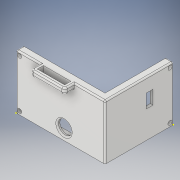
# Autodesk Inventor part: Part1
Saved by Autodesk Inventor 2019 (Build 230136000, 136)
## iProperties
Created: 2019-02-07
Part Number: Part1
Material: ABS Plastic
Document SubType Name: Modeling
Designer: darky
Density: 1.06 g/cm^3
Appearance: Smooth - White
Author: darky
Autodesk Inventor part; units mm, degrees
ref_plane "YZ Plane" through (0, 0, 0) normal (1, 0, 0) x (0, 1, 0)
ref_plane "XZ Plane" through (0, 0, 0) normal (0, 1, 0) x (-1, 0, 0)
ref_plane "XY Plane" through (0, 0, 0) normal (0, 0, 1) x (1, 0, 0)
sketch "Sketch1" plane through (0, 0, 0) normal (0, 0, 1) x (1, 0, 0)
  line L0 (0, 0) -> (65, 0)
  line L1 (65, 0) -> (65, 40)
  line L2 (65, 40) -> (0, 40)
  line L3 (0, 40) -> (0, 0)
  dimension "d0" = 65
  dimension "d1" = 40
  constraints: 8 end point, 2 parallel, 1 horizontal, 1 perpendicular
  measures "d0" distance of L2.end L1.end
  measures "d1" distance of L1.end L0.end
extrude "Extrusion1" add sketch "Sketch1" along normal blind 50
shell "Shell1" thickness 5 removed faces 4 at (43.3333, 40, 16.6667) at (21.6667, 13.3333, 0) at (0, 26.6667, 16.6667) at (21.6667, 0, 16.6667)
sketch "Sketch4" plane through (0, 0, 50) normal (0, 0, 1) x (1, 0, 0)
  line L0 (65, 0) -> (65, 40) projected
  line L1 (65, 0) -> (35, 0)
  line L2 (0, 0) -> (65, 0) projected
  line L3 (35, 0) -> (35, 8)
  circle A0 centre (35, 8) radius 5
  dimension "d17" = 30
  dimension "d18" = 8
  dimension "d19" = 10
  constraints: 4 end point, 1 centre point, 1 coincident, 1 perpendicular, 1 point on line
  measures "d17" distance of L0.start L1.end
  measures "d18" distance of L1.end L3.end
  measures "d19" diameter of A0
extrude "Extrusion4" cut sketch "Sketch4" against normal blind 3
sketch "Sketch5" plane through (0, 0, 50) normal (0, 0, 1) x (1, 0, 0)
  point P0 (0, 0)
sketch "Sketch6" plane through (35, 8, 47) normal (0, 0, 1) x (1, 0, 0)
  circle A0 centre (0, 0) radius 3
  point P0 (-35, -8)
  dimension "d22" = 6
  constraints: 1 centre point
  measures "d22" diameter of A0
extrude "Extrusion5" cut sketch "Sketch6" against normal blind 2
sketch "Sketch7" plane through (0, 0, 50) normal (0, 0, 1) x (1, 0, 0)
  line L0 (0, 0) -> (65, 0) projected
  line L1 (0, 0) -> (5, 0)
  line L2 (5, 0) -> (5, 5)
  line L3 (65, 40) -> (0, 40) projected
  line L4 (5, 5) -> (5, 35)
  line L5 (5, 35) -> (2.5, 37.4495)
  circle A0 centre (2.5, 37.4495) radius 1.9
  dimension "d25" = 5
  dimension "d26" = 5
  dimension "d27" = 30
  dimension "d28" = 3.5
  dimension "d29" = 3.8
  constraints: 8 end point, 2 point on line, 1 centre point, 1 coincident, 1 perpendicular
  measures "d25" distance of L0.start L1.end
  measures "d26" distance of L1.end L2.end
  measures "d27" distance of L2.end L4.end
  measures "d28" distance of L4.end L5.end
  measures "d29" diameter of A0
hole "Hole1" at (2.5, 37.4495, 50) direction (0, 0, -1) diameter 3 depth 9 tip angle 118
sketch "Sketch8" plane through (0, 0, 50) normal (0, 0, 1) x (1, 0, 0)
  line L0 (0, 0) -> (5, 0)
  line L1 (0, 0) -> (65, 0) projected
  line L2 (5, 0) -> (5, 5)
  line L3 (5, 5) -> (2.5505, 2.5)
  circle A0 centre (2.5505, 2.5) radius 1.5
  dimension "d37" = 5
  dimension "d38" = 5
  dimension "d39" = 3.5
  dimension "d40" = 3
  constraints: 6 end point, 1 centre point, 1 coincident, 1 perpendicular, 1 point on line
  measures "d37" distance of L0.start L0.end
  measures "d38" distance of L0.end L2.end
  measures "d39" distance of L2.end L3.end
  measures "d40" diameter of A0
hole "Hole2" at (2.5505, 2.5, 50) direction (0, 0, -1) diameter 3 depth 9 tip angle 118
sketch "Sketch11" plane through (65, 0, 0) normal (1, 0, 0) x (0, 0, -1)
  line L0 (0, 0) -> (-5, 0)
  line L1 (-45, 0) -> (0, 0) projected
  line L2 (-5, 0) -> (-5, 5)
  line L3 (-5, 5) -> (-5, 35)
  line L4 (-5, 35) -> (-2.5251, 37.4749)
  circle A0 centre (-2.5251, 37.4749) radius 1.5
  dimension "d59" = 5
  dimension "d60" = 5
  dimension "d61" = 30
  dimension "d62" = 3.5
  dimension "d63" = 3
  constraints: 8 end point, 2 point on line, 1 centre point, 1 coincident, 1 perpendicular
  measures "d59" distance of L0.start L0.end
  measures "d60" distance of L0.end L2.end
  measures "d61" distance of L2.end L3.end
  measures "d62" distance of L3.end L4.end
  measures "d63" diameter of A0
hole "Hole3" at (65, 37.4749, 2.5251) direction (-1, 0, 0) diameter 3 depth 9 tip angle 118
sketch "Sketch12" plane through (65, 0, 0) normal (1, 0, 0) x (0, 0, -1)
  line L0 (-45, 0) -> (0, 0) projected
  line L1 (0, 0) -> (-5, 0)
  line L2 (-5, 0) -> (-5, 5)
  line L3 (-5, 5) -> (-2.5505, 2.5)
  circle A0 centre (-2.5505, 2.5) radius 1.5
  dimension "d71" = 5
  dimension "d72" = 5
  dimension "d73" = 3.5
  dimension "d74" = 3
  constraints: 6 end point, 1 centre point, 1 coincident, 1 perpendicular, 1 point on line
  measures "d71" distance of L0.end L1.end
  measures "d72" distance of L1.end L2.end
  measures "d73" distance of L2.end L3.end
  measures "d74" diameter of A0
hole "Hole4" at (65, 2.5, 2.5505) direction (-1, 0, 0) diameter 3 depth 9 tip angle 118
sketch "Sketch14" plane through (0, 40, 50) normal (0, 1, 0) x (1, 0, 0)
  line L0 (0, 5) -> (0, 0) projected
  line L1 (0, 5) -> (5, 5)
  line L2 (0, 5) -> (60, 5) projected
  line L3 (5, 5) -> (60, 5)
  line L4 (60, 5) -> (60, 2)
  line L5 (60, 2) -> (5, 2)
  line L6 (5, 2) -> (5, 5)
  point P0 (0, 50)
  dimension "d88" = 5
  dimension "d89" = 3
  constraints: 10 end point, 2 parallel, 1 horizontal, 1 perpendicular, 1 point on line
  measures "d88" distance of L0.start L1.end
  measures "d89" distance of L3.end L4.end
extrude "Extrusion9" cut sketch "Sketch14" against normal blind 40
sketch "Sketch15" plane through (60, 40, 48) normal (0, 0, -1) x (-1, 0, 0)
  line L0 (0, 0) -> (55, 0) projected
  line L1 (55, 0) -> (55, -5)
  line L2 (55, 0) -> (55, -40) projected
  line L3 (55, 0) -> (0, 0)
  line L4 (0, 0) -> (0, -5)
  line L5 (0, -5) -> (55, -5)
  line L6 (55, -5) -> (55, 0)
  line L7 (55, -40) -> (0, -40) projected
  line L8 (0, 0) -> (0, -40) projected
  line L9 (55, -40) -> (0, -40)
  line L10 (0, -40) -> (0, -37.5)
  line L11 (0, -37.5) -> (55, -37.5)
  line L12 (55, -37.5) -> (55, -40)
  point P0 (60, -40)
  dimension "d92" = 5
  dimension "d93" = 2.5
  constraints: 18 end point, 4 parallel, 2 horizontal, 2 perpendicular, 2 point on line
  measures "d92" distance of L0.end L1.end
  measures "d93" distance of L9.end L10.end
extrude "Extrusion10" add sketch "Sketch15" along normal blind 3 contours L0 L1 L5 L4 | L11 L2 L7 L8
sketch "Sketch16" plane through (60, 0, 45) normal (0, 0, -1) x (-1, 0, 0)
  line L0 (55, 35) -> (0, 35) projected
  line L1 (55, 35) -> (58, 35)
  line L2 (58, 35) -> (58, 5)
  line L3 (58, 5) -> (55, 5)
  line L4 (55, 5) -> (55, 35)
  point P0 (60, 0)
  dimension "d96" = 3
  dimension "d97" = 30
  constraints: 8 end point, 2 parallel, 1 horizontal, 1 perpendicular
  measures "d96" distance of L2.end L3.end
  measures "d97" distance of L1.end L2.end
extrude "Extrusion11" cut sketch "Sketch16" against normal blind 3
sketch "Sketch17" plane through (0, 0, 0) normal (0, 0, -1) x (-1, 0, 0)
  line L0 (-60, 35) -> (-63, 35)
  line L1 (-63, 35) -> (-63, 5)
  line L2 (-63, 5) -> (-60, 5)
  line L3 (-60, 5) -> (-60, 35)
  point P0 (0, 0)
  dimension "d100" = 3
  dimension "d101" = 30
  constraints: 8 end point, 2 parallel, 1 horizontal, 1 perpendicular
  measures "d100" distance of L2.end L1.end
  measures "d101" distance of L1.end L0.end
extrude "Extrusion12" cut sketch "Sketch17" against normal blind 45
sketch "Sketch18" plane through (63, 5, 0) normal (-1, 0, 0) x (0, 0, 1)
  line L0 (0, 30) -> (2, 30)
  line L1 (2, 30) -> (2, 0)
  line L2 (2, 0) -> (0, 0)
  line L3 (0, 0) -> (0, 30)
  point P0 (0, -5)
  dimension "d104" = 2
  dimension "d105" = 30
  constraints: 8 end point, 2 parallel, 1 horizontal, 1 perpendicular
  measures "d104" distance of L1.end L2.end
  measures "d105" distance of L0.end L1.end
extrude "Extrusion13" add sketch "Sketch18" along normal blind 3
sketch "Sketch19" plane through (60, 0, 0) normal (-1, 0, 0) x (0, 0, 1)
  line L0 (0, 0) -> (0, 40) projected
  line L1 (0, 40) -> (5, 40)
  line L2 (0, 40) -> (50, 40) projected
  line L3 (5, 40) -> (5, 35)
  line L4 (45, 40) -> (45, 0) projected
  line L5 (5, 35) -> (45, 35)
  line L6 (45, 35) -> (45, 38)
  line L7 (45, 38) -> (5, 38)
  line L8 (5, 38) -> (5, 35)
  dimension "d108" = 5
  dimension "d109" = 5
  dimension "d110" = 3
  constraints: 12 end point, 2 parallel, 2 point on line, 1 horizontal, 1 perpendicular, 1 vertical
  measures "d108" distance of L0.end L1.end
  measures "d109" distance of L1.end L3.end
  measures "d110" distance of L6.end L5.end
extrude "Extrusion14" add sketch "Sketch19" against normal blind 3 contours L7 L4 L5 L3
sketch "Sketch20" plane through (60, 0, 0) normal (-1, 0, 0) x (0, 0, 1)
  line L0 (0, 40) -> (50, 40) projected
  line L1 (0, 40) -> (5, 40)
  line L2 (5, 40) -> (5, 35)
  line L3 (5, 35) -> (45, 35)
  line L4 (45, 35) -> (45, 38)
  line L5 (45, 38) -> (5, 38)
  line L6 (5, 38) -> (5, 35)
  point P0 (0, 0)
  dimension "d113" = 5
  dimension "d114" = 5
  dimension "d115" = 3
  constraints: 12 end point, 2 parallel, 2 perpendicular, 1 horizontal, 1 point on line
  measures "d113" distance of L0.start L1.end
  measures "d114" distance of L1.end L2.end
  measures "d115" distance of L4.end L3.end
extrude "Extrusion15" add sketch "Sketch20" against normal blind 3
sketch "Sketch21" plane through (60, 5, 45) normal (0, 1, 0) x (1, 0, 0)
  line L0 (3, 43) -> (0, 43) projected
  line L1 (0, 43) -> (0, 40)
  line L2 (0, 0) -> (0, 43) projected
  line L3 (3, 43) -> (3, 0) projected
  line L4 (0, 40) -> (3, 40)
  line L5 (3, 40) -> (3, 0)
  line L6 (3, 0) -> (0, 0)
  line L7 (0, 0) -> (0, 40)
  point P0 (-60, 45)
  dimension "d118" = 3
  dimension "d119" = 3
  dimension "d120" = 40
  constraints: 10 end point, 2 parallel, 1 horizontal, 1 perpendicular, 1 point on line
  measures "d118" distance of L0.end L1.end
  measures "d119" distance of L3.end L6.end
  measures "d120" distance of L4.end L3.end
extrude "Extrusion16" cut sketch "Sketch21" against normal blind 3 contours L3 L6 L2 L4
sketch "Sketch22" plane through (60, 35, 45) normal (0, -1, 0) x (1, 0, 0)
  line L0 (0, -43) -> (0, -40)
  line L1 (3, -43) -> (3, 0) projected
  line L2 (0, -40) -> (3, -40)
  line L3 (3, -40) -> (3, 0)
  line L4 (3, 0) -> (0, 0)
  line L5 (0, 0) -> (0, -40)
  point P0 (-60, -45)
  dimension "d123" = 3
  dimension "d124" = 40
  constraints: 10 end point, 2 parallel, 1 horizontal, 1 perpendicular, 1 vertical
  measures "d123" distance of L0.start L0.end
  measures "d124" distance of L1.end L2.end
extrude "Extrusion17" cut sketch "Sketch22" against normal blind 3
sketch "Sketch23" plane through (60, 35, 45) normal (0, -1, 0) x (1, 0, 0)
  line L0 (0, 0) -> (-58, 0) projected
  line L1 (-58, 3) -> (0, 3) projected
  line L2 (0, 0) -> (-55, 0)
  line L3 (-55, 0) -> (-55, 3)
  line L4 (-55, 3) -> (0, 3)
  line L5 (0, 3) -> (0, 0)
  point P0 (-60, -45)
  dimension "d127" = 55
  constraints: 8 end point, 2 parallel, 1 horizontal, 1 perpendicular, 1 point on line
  measures "d127" distance of L3.end L4.end
extrude "Extrusion18" cut sketch "Sketch23" against normal blind 3
fillet "Fillet2" radius 1 6 edges at (0, 0, 47.5) (0, 40, 47.5) (0, 20, 50) (62.5, 40, 0) (62.5, 0, 0) (65, 20, 0)
fillet "Fillet3" radius 1 1 edges at (30, 8, 50)
sketch "Sketch26" plane through (0, 0, 50) normal (0, 0, 1) x (1, 0, 0)
  line L0 (0, 0) -> (0, 40)
  line L1 (0, 39) -> (0, 1) projected
  line L2 (1, 39) -> (64, 39) projected
  line L3 (0, 40) -> (30, 40)
  line L4 (60, 40) -> (1, 40) projected
  line L5 (30, 40) -> (17.5, 40)
  line L6 (17.5, 40) -> (42.5, 40)
  line L7 (42.5, 40) -> (42.5, 35)
  line L8 (42.5, 35) -> (17.5, 35)
  line L9 (17.5, 35) -> (17.5, 40)
  dimension "d148" = 40
  dimension "d150" = 30
  dimension "d151" = 12.5
  dimension "d152" = 25
  dimension "d153" = 5
  constraints: 14 end point, 2 parallel, 2 point on line, 1 collinear, 1 horizontal, 1 perpendicular
  measures "d148" distance of L0.start L0.end
  measures "d150" distance of L0.end L3.end
  measures "d151" distance of L3.end L5.end
  measures "d152" distance of L7.end L8.end
  measures "d153" distance of L6.end L7.end
extrude "Extrusion21" add sketch "Sketch26" along normal blind 7
sketch "Sketch27" plane through (1, 40, 45) normal (0, 1, 0) x (1, 0, 0)
  line L0 (41.5, -5) -> (16.5, -5) projected
  line L1 (16.5, -5) -> (19, -5)
  line L2 (19, -5) -> (39, -5)
  line L3 (39, -5) -> (39, -9.5)
  line L4 (39, -9.5) -> (19, -9.5)
  line L5 (19, -9.5) -> (19, -5)
  point P0 (-1, 45)
  dimension "d156" = 2.5
  dimension "d157" = 20
  dimension "d158" = 4.5
  constraints: 10 end point, 2 parallel, 1 horizontal, 1 perpendicular, 1 point on line
  measures "d156" distance of L0.end L1.end
  measures "d157" distance of L3.end L4.end
  measures "d158" distance of L2.end L3.end
extrude "Extrusion22" cut sketch "Sketch27" against normal blind 5
fillet "Fillet5" radius 1 6 edges at (0.2929, 39.7071, 49.7071) (9.25, 40, 50) (53.75, 40, 50) (64.7071, 39.7071, 0.2929) (65, 40, 25.5) (65, 20, 50)
fillet "Fillet6" radius 1 3 edges at (30, 40, 57) (17.5, 40, 53) (42.5, 40, 53)
fillet "Fillet7" radius 2 7 edges at (30, 35, 57) (17.7929, 39.7071, 56.7071) (17.5, 37, 57) (17.5, 35, 53.5) (42.5, 35, 53.5) (42.2071, 39.7071, 56.7071) (42.5, 37, 57)
sketch "Sketch28" plane through (65, 0, 49) normal (1, 0, 0) x (0, 0, -1)
  point P0 (49, 0)
sketch "Sketch29" plane through (65, 0, 49) normal (1, 0, 0) x (0, 0, -1)
  line L0 (44, 30) -> (44, 20) projected
  line L1 (44, 30) -> (34, 30)
  line L2 (34, 30) -> (29, 30)
  line L3 (29, 30) -> (29, 20)
  line L4 (29, 20) -> (34, 20)
  line L5 (34, 20) -> (34, 30)
  point P0 (49, 0)
  dimension "d164" = 10
  dimension "d165" = 5
  dimension "d166" = 10
  constraints: 10 end point, 2 horizontal, 2 parallel, 1 perpendicular
  measures "d164" distance of L0.start L1.end
  measures "d165" distance of L4.end L3.end
  measures "d166" distance of L3.end L2.end
extrude "Extrusion23" cut sketch "Sketch29" against normal blind 2
body "Solid1"
